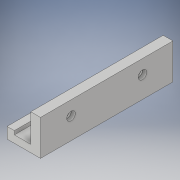
# Autodesk Inventor part: bottomSpacer
Saved by Autodesk Inventor 2017 (Build 210142000, 142)
## iProperties
Created: 2022-11-19
Part Number: bottomSpacer
Material: Generic
Document SubType Name: Modeling
Designer: khonsu
Density: 1 g/cm^3
Appearance: Default
Author: khonsu
Autodesk Inventor part; units mm, degrees
ref_plane "YZ Plane" through (0, 0, 0) normal (1, 0, 0) x (0, 1, 0)
ref_plane "XZ Plane" through (0, 0, 0) normal (0, 1, 0) x (-1, 0, 0)
ref_plane "XY Plane" through (0, 0, 0) normal (0, 0, 1) x (1, 0, 0)
sketch "Sketch1" plane through (0, 0, 0) normal (0, 0, 1) x (1, 0, 0)
  line L0 (0, 0) -> (0, 4.5)
  line L1 (0, 0) -> (0, 4.5)
  line L2 (0, 4.5) -> (3, 4.5)
  line L3 (0, 4.5) -> (3, 4.5)
  line L4 (3, 4.5) -> (3, 3)
  line L5 (3, 4.5) -> (3, 3)
  line L6 (3, 3) -> (9.7, 3)
  line L7 (3, 3) -> (9.7, 3)
  line L8 (9.7, 3) -> (9.7, 14.544)
  line L9 (9.7, 3) -> (9.7, 14.544)
  line L10 (13.7, 14.544) -> (9.7, 14.544)
  line L11 (9.7, 14.544) -> (13.7, 14.544)
  line L12 (13.7, 14.544) -> (13.7, 0)
  line L13 (13.7, 0) -> (0, 0)
  line L14 (13.7, 0) -> (0, 0)
  point P0 (13.7, 167.0499)
  constraints: 30 end point, 7 collinear, 1 perpendicular
extrude "Extrusion1" add sketch "Sketch1" along normal blind 54.3
sketch "Sketch2" plane through (9.7, 3, 0) normal (-1, 0, 0) x (0, 0, 1)
  circle A0 centre (12.5, 5.772) radius 1.75
  circle A1 centre (41.8, 5.772) radius 1.75
  line L0 (0, 11.544) -> (0, 0) projected
  line L1 (54.3, 11.544) -> (54.3, 0) projected
  point P0 (0, -3)
  dimension "d2" = 3.5
  dimension "d3" = 3.5
  dimension "d4" = 12.5
  dimension "d5" = 12.5
  constraints: 2 centre point
  measures "d2" diameter of A0
  measures "d3" diameter of A1
  measures "d4" distance from line of L0 A0.centre
  measures "d5" distance from line of L1 A1.centre
extrude "Extrusion2" cut sketch "Sketch2" against normal blind 54.3
chamfer "Chamfer1" distance 2.4 angle 45 2 edges at (9.7, 8.772, 10.75) (9.7, 8.772, 40.05)
equation "\"d5\" = d4"
body "Solid1"
